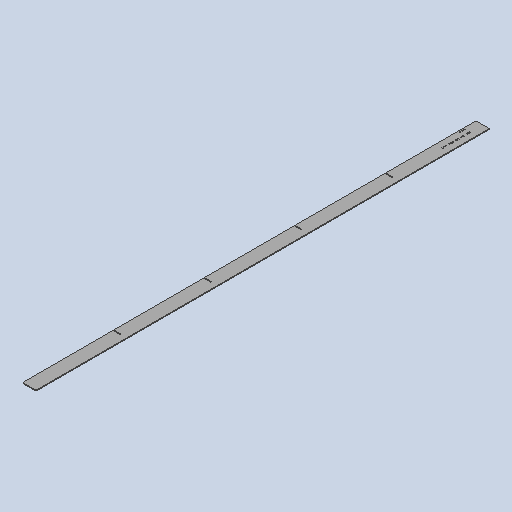
# Autodesk Inventor part: MSC 604 RIB CONE EXIT BACK
Saved by Autodesk Inventor 2025 (Build 290162010, 162A)
## iProperties
Created: 2024-08-26
Part Number: MSC 604 RIB CONE EXIT BACK
Material: Stainless Steel
Document SubType Name: Sheet Metal
Designer: pokla
Density: 8 g/cm^3
Sheet Metal Rule: AISI304 3mm Die 32
Appearance: Default
Stock Number: МОО 604 шпангоут конус выход корма
Mass: 2032.14 g
Surface Area: 1804.54 cm^2
Volume: 254.018 cm^3
Flat Pattern Width: 5 cm
Flat Pattern Length: 170 cm
Flat Pattern Area: 850 cm^2
Sheet Metal Width: 50,000 mm
Sheet Metal Length: 1700,000 mm
Sheet Metal Area: 85000,000 mm^2
Author: pokla
Autodesk Inventor part; units mm, degrees
ref_plane "YZ Plane" through (0, 0, 0) normal (1, 0, 0) x (0, 1, 0)
ref_plane "XZ Plane" through (0, 0, 0) normal (0, 1, 0) x (-1, 0, 0)
ref_plane "XY Plane" through (0, 0, 0) normal (0, 0, 1) x (1, 0, 0)
sketch "Sketch1" plane through (0, 0, 0) normal (0, 0, 1) x (1, 0, 0)
  line L0 (-25, 0) -> (25, 0)
  line L1 (25, 0) -> (25, -1700)
  line L2 (25, -1700) -> (-25, -1700)
  line L3 (-25, -1700) -> (-25, 0)
  point P0 (0, 0)
  point P1 (0, 0)
  point P2 (-25, -1153.2713)
  dimension "d0" = 50
  dimension "d1" = 1700
  measures "d0" distance of L0.start L0.end
  measures "d1" distance of L2.end L0.start
extrude "Plate1" add sketch "Sketch1" along normal mid plane 3
sketch "Sketch2" plane through (0, 0, 1.5) normal (0, 0, 1) x (1, 0, 0)
  line L0 (-25, -1021.5) -> (1, -1021.5)
  line L1 (1, -1021.5) -> (1, -1018.5)
  line L2 (1, -1018.5) -> (-25, -1018.5)
  line L3 (-25, -1018.5) -> (-25, -1021.5)
  line L4 (-25, -1700) -> (-25, 0) projected
  line L5 (-25, -1361.5) -> (1, -1361.5)
  line L6 (1, -1361.5) -> (1, -1358.5)
  line L7 (1, -1358.5) -> (-25, -1358.5)
  line L8 (-25, -1358.5) -> (-25, -1361.5)
  line L9 (-25, -681.5) -> (1, -681.5)
  line L10 (1, -681.5) -> (1, -678.5)
  line L11 (1, -678.5) -> (-25, -678.5)
  line L12 (-25, -678.5) -> (-25, -681.5)
  line L13 (-25, -341.5) -> (1, -341.5)
  line L14 (1, -341.5) -> (1, -338.5)
  line L15 (1, -338.5) -> (-25, -338.5)
  line L16 (-25, -338.5) -> (-25, -341.5)
  point P0 (0, 0)
  point P1 (-25, -1020)
  point P2 (-25, -850)
  point P3 (-25, -1360)
  point P4 (-25, -680)
  point P5 (-25, -850)
  point P6 (-25, -340)
  point P7 (-25, -338.5)
  point P8 (-25, -341.5)
  point P9 (-25, -678.5)
  point P10 (-25, -681.5)
  point P11 (-25, -1358.5)
  point P12 (-25, -1361.5)
  dimension "d15" = 26
  dimension "d16" = 3
  dimension "d17" = 170
  dimension "d20" = 26
  dimension "d21" = 3
  dimension "d22" = 340
  dimension "d23" = 26
  dimension "d24" = 3
  dimension "d25" = 170
  dimension "d26" = 340
  dimension "d27" = 3
  dimension "d28" = 26
  constraints: 32 end point, 8 parallel, 6 midpoint, 4 horizontal, 4 perpendicular, 4 point on line
  measures "d15" distance of L0.start L0.end
  measures "d16" distance of L2.end L0.start
  measures "d17" distance of point (-25, -850) point (-25, -1020)
  measures "d20" distance of L5.start L5.end
  measures "d21" distance of L7.end L5.start
  measures "d22" distance of point (-25, -1020) point (-25, -1360)
  measures "d23" distance of L9.start L9.end
  measures "d24" distance of L9.end L10.end
  measures "d25" distance of point (-25, -850) point (-25, -680)
  measures "d26" distance of point (-25, -680) point (-25, -340)
  measures "d27" distance of L13.end L14.end
  measures "d28" distance of L13.start L13.end
extrude "Extrusion1" cut sketch "Sketch2" against normal through all
fillet "Corner Round3" radius 6 2 edges at (-25, 0, 0) (-25, -1700, 0)
sketch "Sketch3" plane through (0, 0, 1.5) normal (0, 0, 1) x (1, 0, 0)
  line L0 (-5.1757, -47.7196) -> (3.8521, -47.7196) construction
  line L1 (3.8521, -47.7196) -> (3.8521, -156.6657) construction
  line L2 (3.8521, -156.6657) -> (-5.1757, -156.6657) construction
  line L3 (-5.1757, -156.6657) -> (-5.1757, -47.7196) construction
  point P0 (0, 0)
  constraints: 2 other
mark "Mark1"
equation "\"d17\" = d25"
equation "\"d20\" = d15"
equation "\"d21\" = d16"
equation "\"d22\" = d26"
equation "\"d23\" = d15"
equation "\"d24\" = d16"
equation "\"d27\" = d24"
equation "\"d28\" = d23"
equation "\"d2\" = Thickness"
equation "\"BendReliefWidth\" = Thickness"
equation "\"BendReliefDepth\" = 0.5 * Thickness"
equation "\"CornerReliefSize\" = 4 * Thickness"
equation "\"MinimumRemnant\" = 2 * Thickness"
equation "\"TransitionRadius\" = BendRadius"
equation "\"JacobiRadiusSize\" = BendRadius"
equation "\"GapSize\" = Thickness"
equation "\"Thickness\" = 3"
equation "\"BendRadius\" = 5"
body "Solid1"
